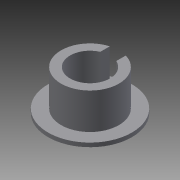
# Autodesk Inventor part: slip_ring_i_2
Saved by Autodesk Inventor 2015 (Build 190159000, 159)
## iProperties
Created: 2017-12-06
Part Number: slip_ring_i_2
Material: Generic
Document SubType Name: Modeling
Designer: Anshul
Density: 1 g/cm^3
Appearance: Default
Author: Anshul
Autodesk Inventor part; units mm, degrees
ref_plane "YZ Plane" through (0, 0, 0) normal (1, 0, 0) x (0, 1, 0)
ref_plane "XZ Plane" through (0, 0, 0) normal (0, 1, 0) x (-1, 0, 0)
ref_plane "XY Plane" through (0, 0, 0) normal (0, 0, 1) x (1, 0, 0)
sketch "Sketch1" plane through (0, 0, 0) normal (0, 1, 0) x (-1, 0, 0)
  circle A0 centre (0, 0) radius 7.25
  arc A1 (2, -4.5826) -> (-2, -4.5826) centre (0, 0) ccw
  line L0 (0, 0) -> (2, 0)
  line L1 (0, 0) -> (2, 0)
  line L2 (2, 0) -> (2, -6.9687)
  line L3 (0, 0) -> (-2, 0)
  line L4 (-2, 0) -> (-2, -6.9687)
  circle A2 centre (0, 0) radius 10.5
  dimension "d0" = 14.5
  dimension "d1" = 10
  dimension "d2" = 2
  dimension "d3" = 2
  dimension "d4" = 2
  dimension "d5" = 21
  constraints: 10 end point, 4 point on circle, 3 centre point, 3 coincident, 3 point on line, 2 horizontal, 2 perpendicular
  measures "d0" diameter of A0
  measures "d1" diameter of A1
  measures "d2" distance of L0.start L0.end
  measures "d3" distance of L0.start L0.end
  measures "d4" distance of L0.start L3.end
  measures "d5" diameter of A2
extrude "Extrusion1" add sketch "Sketch1" along normal blind 10 contours A0 L2 A1 L4
extrude "Extrusion2" add sketch "Sketch1" along normal blind 1
body "Solid1"
